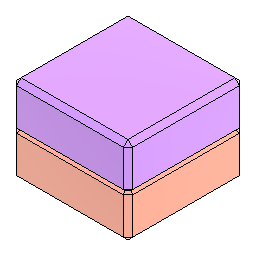
JE_RingBox (Autodesk Fusion 360 design; units mm, degrees)
Autodesk Fusion 360 part; units mm, degrees
ref_plane "WorkPlane1" through (0, 0, 0) normal (0, 0, 1) x (1, 0, 0)
ref_plane "WorkPlane1" through (0, 0, 0) normal (0, 1, 0) x (0, 0, 1) in component "RingBox_Bottom"
sketch "RB_Bottom" plane through (0, 0, 0) normal (0, 1, 0) x (1, 0, 0) in component "RingBox_Bottom"
  line L0 (25.4, 0) -> (76.2, 0)
  line L1 (76.2, 0) -> (76.2, 19.05)
  line L2 (76.2, 19.05) -> (25.4, 19.05)
  line L3 (25.4, 19.05) -> (25.4, 0)
  point P0 (25.4, 0)
  dimension "Z_RB_Bottom_Orig" = 0
  dimension "X_RB_Bottom_Orig" = 25.4
  dimension "RB_Bottom_Thickness" = 19.05
  dimension "RB_Bottom_Width" = 50.8
  constraint horizontal L0
  constraint vertical L1
  constraint horizontal L2
  constraint vertical L3
  constraint coincident P0 L0.start
  measures "Z_RB_Bottom_Orig" vertical distance of origin L0.start
  measures "X_RB_Bottom_Orig" horizontal distance of origin L0.start
  measures "RB_Bottom_Thickness" distance of P0 L2.end
  measures "RB_Bottom_Width" distance of L1.end L2.end
extrude "Extrude1" add sketch "RB_Bottom" along normal blind 50.8 makes body 1 in component "RingBox_Bottom"
ref_plane "WorkPlane1" through (0, 0, 0) normal (0, 1, 0) x (0, 0, 1) in component "RingBox_Top"
sketch "Sketch1" plane through (0, 0, 0) normal (0, 1, 0) x (1, 0, 0) in component "RingBox_Top"
  line L0 (25.4, 0) -> (76.2, 0)
  line L1 (76.2, 0) -> (76.2, -19.05)
  line L2 (76.2, -19.05) -> (25.4, -19.05)
  line L3 (25.4, -19.05) -> (25.4, 0)
  point P0 (25.4, 0)
  dimension "Z_RB_Top_Orig" = 0
  dimension "X_RB_Top_Orig" = 25.4
  dimension "RB_Top_Width" = 50.8
  dimension "RB_Top_Thickness" = 19.05
  constraint horizontal L0
  constraint vertical L1
  constraint horizontal L2
  constraint vertical L3
  constraint coincident P0 L0.start
  measures "Z_RB_Top_Orig" vertical distance of origin L0.start
  measures "X_RB_Top_Orig" horizontal distance of origin L0.start
  measures "RB_Top_Width" distance of P0 L0.end
  measures "RB_Top_Thickness" distance of P0 L2.end
extrude "Extrude1'" add sketch "Sketch1" along normal blind 50.8 separate body makes body 2 in component "RingBox_Top"
ref_plane "WorkPlane2" through (0, 0, 0) normal (0, 0, 1) x (1, 0, 0) in component "RingBox_Bottom"
sketch "RBB_Holes" plane through (0, 0, 0) normal (0, 0, 1) x (1, 0, 0) in component "RingBox_Bottom"
  circle A0 centre (50.8, 25.4) radius 12.7
  line L0 (25.4, 50.8) -> (76.2, 50.8)
  line L1 (25.4, 0) -> (25.4, 50.8)
  circle A1 centre (34.925, 43.8) radius 4.175
  circle A2 centre (66.675, 43.8) radius 4.175
  point P0 (50.8, 25.4)
  point P1 (34.925, 43.8)
  point P2 (66.675, 43.8)
  dimension "Y_RBB_Holes_Orig" = -25.4
  dimension "X_RBB_Holes_Orig" = 50.8
  dimension "RBBH_Ring_Diameter" = 25.4
  dimension "Hinge1_Y_Offset" = 18.4
  dimension "RBB_DistanceBTWParts1" = 15.875
  dimension "Hinge2_Y_Offset" = 18.4
  dimension "RBB_DistanceBTWParts2" = 15.875
  dimension "RBBH_Barrel1_Diameter" = 8.35
  dimension "RBBH_Barrel2_Diameter" = 8.35
  constraint coincident P0 A0.centre
  constraint coincident P1 A1.centre
  constraint coincident P2 A2.centre
  measures "Y_RBB_Holes_Orig" vertical distance of P0 origin
  measures "X_RBB_Holes_Orig" horizontal distance of P0 origin
  measures "RBBH_Ring_Diameter" diameter of A0
  measures "Hinge1_Y_Offset" vertical distance of P0 P1
  measures "RBB_DistanceBTWParts1" horizontal distance of P0 A1.centre
  measures "Hinge2_Y_Offset" vertical distance of P0 P2
  measures "RBB_DistanceBTWParts2" horizontal distance of P0 P2
  measures "RBBH_Barrel1_Diameter" diameter of A1
  measures "RBBH_Barrel2_Diameter" diameter of A2
extrude "Extrude2" cut sketch "RBB_Holes" along normal mid plane 16 contours A1 | A2 bodies 1 in component "RingBox_Bottom"
chamfer "Chamfer1" distance 2 angle 45 8 edges at (76.2, 50.8, -9.525) (25.4, 50.8, -9.525) (25.4, 0, -9.525) (50.8, 50.8, -19.05) (25.4, 25.4, -19.05) (50.8, 0, -19.05) (76.2, 25.4, -19.05) (76.2, 0, -9.525) on bodies 1 in component "RingBox_Bottom"
chamfer "Chamfer1'" distance 2 angle 45 8 edges at (76.2, 25.4, 19.05) (50.8, 0, 19.05) (76.2, 0, 9.525) (76.2, 50.8, 9.525) (25.4, 50.8, 9.525) (25.4, 0, 9.525) (25.4, 25.4, 19.05) (50.8, 50.8, 19.05) on bodies 2 in component "RingBox_Top"
chamfer "Chamfer2" distance 1 angle 45 8 edges at (25.4, 25.4, 0) (50.8, 0, 0) (76.2, 25.4, 0) (50.8, 50.8, 0) (75.2, 49.8, 0) (26.4, 49.8, 0) (26.4, 1, 0) (75.2, 1, 0) on bodies 1 in component "RingBox_Bottom"
chamfer "Chamfer2'" distance 1 angle 45 8 edges at (25.4, 25.4, 0) (26.4, 49.8, 0) (50.8, 50.8, 0) (75.2, 49.8, 0) (76.2, 25.4, 0) (75.2, 1, 0) (26.4, 1, 0) (50.8, 0, 0) on bodies 2 in component "RingBox_Top"
extrude "Extrude2'" cut sketch "RBB_Holes" along normal blind 8 contours A1 | A2 bodies 2 in component "RingBox_Top"
extrude "Extrude3" cut sketch "RBB_Holes" against normal blind 15.875 contours A0 bodies 1 in component "RingBox_Bottom"
extrude "Extrude3'" cut sketch "RBB_Holes" along normal blind 6.35 contours A0 bodies 2 in component "RingBox_Top"
component "RingBox_Top" placed x (1, 0, 0) y (0, 1, 0) z (0, 0, 1) at (0, 0, 0)
component "RingBox_Bottom" placed x (1, 0, 0) y (0, 1, 0) z (0, 0, 1) at (0, 0, 0)
equation "Shared_Kerf = 0.125 in"
equation "Z_RingBox_Orig = 0 in"
equation "Shared_Material_Thickness = 2 in"
equation "Y_RB_Bottom_Orig = 0 in"
equation "RB_Bottom_Thickness = Shared_Total_Height / 2"
equation "RB_Bottom_Width = Shared_Material_Thickness"
equation "RB_Bottom_Length = Shared_Material_Thickness"
equation "Y_RB_Top_Orig = Y_RB_Bottom_Orig"
equation "RB_Top_Width = Shared_Material_Thickness"
equation "RB_Top_Thickness = Shared_Total_Height / 2" comment "make sure to incude kerf when cutting stock"
equation "RB_Top_Length = Shared_Material_Thickness"
equation "Z_RBB_Holes_Orig = Z_RB_Bottom_Orig"
equation "Y_RBB_Holes_Orig = -( Y_RB_Bottom_Orig + ( RB_Bottom_Length / 2 ) )"
equation "X_RBB_Holes_Orig = X_RB_Bottom_Orig + ( RB_Bottom_Width / 2 )"
equation "Hinge_Y_Offset = 7 mm"
equation "Hinge1_Y_Offset = ( RB_Bottom_Length / 2 ) - Hinge_Y_Offset"
equation "Hinge_DistBTWParts = 1.25 in"
equation "RBB_DistanceBTWParts1 = Hinge_DistBTWParts / 2"
equation "Hinge2_Y_Offset = ( RB_Bottom_Length / 2 ) - Hinge_Y_Offset"
equation "RBB_DistanceBTWParts2 = Hinge_DistBTWParts / 2"
equation "RBBH_Barrel1_Diameter = Shared_Barrel_Diameter"
equation "RBBH_Barrel2_Diameter = Shared_Barrel_Diameter"
equation "Shared_Barrel_Diameter = 8.35 mm"
equation "RBH_Hinge_Depth = Shared_Hinge_Depth"
equation "External_Chamfer = 2 mm"
equation "Internal_Chamfer = 1 mm"
equation "RTH_Hinge_Depth = Shared_Hinge_Depth"
equation "RBBH_Ring_Depth = -( RB_Bottom_Thickness - 0.125 in )"
equation "RBTH_Ring_Depth = 0.25 in"
equation "Shared_Total_Height = 1.5 in"
equation "Shared_Hinge_Depth = 8 mm"
